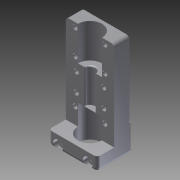
# Autodesk Inventor part: Z move left
Saved by Autodesk Inventor 2012 (Build 160160000, 160)
## iProperties
Created: 2013-02-04
Part Number: Z move left
Material: Default
Document SubType Name: Modeling
Designer: mce
Density: 1 g/cm^3
Mass: 50.5221 g
Surface Area: 165.701 cm^2
Volume: 50.5221 cm^3
Author: mce
Autodesk Inventor part; units mm, degrees
ref_plane "YZ Plane" through (0, 0, 0) normal (1, 0, 0) x (0, 1, 0)
ref_plane "XZ Plane" through (0, 0, 0) normal (0, 1, 0) x (-1, 0, 0)
ref_plane "XY Plane" through (0, 0, 0) normal (0, 0, 1) x (1, 0, 0)
sketch "Sketch1" plane through (0, 0, 0) normal (0, 0, 1) x (1, 0, 0)
  line L0 (0, 0) -> (42.4, 0)
  line L1 (42.4, 0) -> (42.4, 30)
  line L2 (42.4, 30) -> (0, 30)
  line L3 (0, 30) -> (0, 0)
  circle A0 centre (21.2, 15) radius 4.5
  dimension "d0" = 42.4
  dimension "d1" = 30
  dimension "d2" = 21.2
  dimension "d3" = 15
  dimension "d4" = 9
  constraints: 8 end point, 2 horizontal, 2 vertical, 1 centre point
  measures "d0" distance of L0.start L0.end
  measures "d1" distance of L2.end L0.start
  measures "d2" distance from line of L3 A0.centre
  measures "d3" distance from line of L0 A0.centre
  measures "d4" diameter of A0
extrude "Extrusion1" add sketch "Sketch1" along normal blind 90
sketch "Sketch2" plane through (0, 0, 90) normal (0, 0, 1) x (1, 0, 0)
  circle A0 centre (21.2, 15) radius 4.5 projected
  circle A1 centre (21.2, 15) radius 10.5
  dimension "d7" = 21
  constraints: 1 centre point, 1 coincident
  measures "d7" diameter of A1
sketch "Sketch3" plane through (0, 0, 0) normal (0, 0, -1) x (-1, 0, 0)
  circle A0 centre (-21.2, 15) radius 4.5 projected
  circle A1 centre (-21.2, 15) radius 10.5
  dimension "d8" = 21
  constraints: 1 centre point, 1 coincident
  measures "d8" diameter of A1
extrude "Extrusion2" cut sketch "Sketch2" against normal blind 30
sketch "Sketch4" plane through (0, 0, 0) normal (0, -1, 0) x (1, 0, 0)
  line L0 (0, 0) -> (42.4, 0) projected
  line L1 (42.4, 0) -> (42.4, 90) projected
  line L2 (0, 90) -> (42.4, 90)
  line L3 (42.4, 90) -> (42.4, 12)
  line L4 (42.4, 12) -> (0, 12)
  line L5 (0, 12) -> (0, 90)
  dimension "d11" = 12
  constraints: 8 end point, 1 point on line
  measures "d11" distance between parallel lines of L4 L0
extrude "Extrusion3" cut sketch "Sketch4" against normal blind 15
extrude "Extrusion4" cut sketch "Sketch3" against normal blind 30
sketch "Sketch5" plane through (0, 0, 0) normal (0, -1, 0) x (1, 0, 0)
  line L0 (0, 0) -> (42.4, 0) projected
  circle A0 centre (8.2, 4) radius 2.1
  circle A1 centre (34.2, 4) radius 2.1
  circle A2 centre (34.2, 26) radius 2.1
  circle A3 centre (8.2, 26) radius 2.1
  circle A4 centre (8.2, 86) radius 2.1
  circle A5 centre (8.2, 64) radius 2.1
  circle A6 centre (34.2, 86) radius 2.1
  circle A7 centre (34.2, 64) radius 2.1
  line L1 (0, 12) -> (0, 90) projected
  line L2 (8.2, 75.2078) -> (8.2, -13.8243) construction
  line L3 (34.2, 77.256) -> (34.2, -15.4673) construction
  line L4 (42.4, 90) -> (42.4, 12) construction
  line L5 (0, 90) -> (10.7, 90) construction
  line L6 (31.7, 90) -> (42.4, 90) construction
  dimension "d16" = 4.2
  dimension "d18" = 8.2
  dimension "d19" = 4
  dimension "d20" = 22
  dimension "d21" = 4
  dimension "d22" = 22
  dimension "d23" = 8.2
  dimension "d24" = 4
  dimension "d25" = 22
  dimension "d26" = 4
  dimension "d27" = 22
  constraints: 8 centre point, 8 point on line, 7 equal radius, 4 end point, 1 vertical
  measures "d16" diameter of A4
  measures "d18" distance between parallel lines of L3 L4
  measures "d19" distance from line of A4.centre L5
  measures "d20" distance of A4.centre A5.centre
  measures "d21" distance from line of L6 A6.centre
  measures "d22" distance of A7.centre A6.centre
  measures "d23" distance between parallel lines of L1 L2
  measures "d24" distance from line of L0 A0.centre
  measures "d25" distance of A3.centre A0.centre
  measures "d26" distance from line of L0 A1.centre
  measures "d27" distance of A2.centre A1.centre
extrude "Extrusion5" cut sketch "Sketch5" against normal through all
sketch "Sketch6" plane through (0, 30, 0) normal (0, 1, 0) x (1, 0, 0)
  circle A0 centre (34.2, -64) radius 2.1 projected
  circle A1 centre (34.2, -86) radius 2.1 projected
  circle A2 centre (8.2, -64) radius 2.1 projected
  circle A3 centre (8.2, -86) radius 2.1 projected
  line L0 (12.2992, -64) -> (10.2496, -67.55)
  line L1 (10.2496, -67.55) -> (6.1504, -67.55)
  line L2 (6.1504, -67.55) -> (4.1008, -64)
  line L3 (4.1008, -64) -> (6.1504, -60.45)
  line L4 (6.1504, -60.45) -> (10.2496, -60.45)
  line L5 (10.2496, -60.45) -> (12.2992, -64)
  line L6 (38.2992, -64) -> (36.2496, -67.55)
  line L7 (36.2496, -67.55) -> (32.1504, -67.55)
  line L8 (32.1504, -67.55) -> (30.1008, -64)
  line L9 (30.1008, -64) -> (32.1504, -60.45)
  line L10 (32.1504, -60.45) -> (36.2496, -60.45)
  line L11 (36.2496, -60.45) -> (38.2992, -64)
  line L12 (38.2992, -86) -> (36.2496, -89.55)
  line L13 (36.2496, -89.55) -> (32.1504, -89.55)
  line L14 (32.1504, -89.55) -> (30.1008, -86)
  line L15 (30.1008, -86) -> (32.1504, -82.45)
  line L16 (32.1504, -82.45) -> (36.2496, -82.45)
  line L17 (36.2496, -82.45) -> (38.2992, -86)
  line L18 (12.2992, -86) -> (10.2496, -89.55)
  line L19 (10.2496, -89.55) -> (6.1504, -89.55)
  line L20 (6.1504, -89.55) -> (4.1008, -86)
  line L21 (4.1008, -86) -> (6.1504, -82.45)
  line L22 (6.1504, -82.45) -> (10.2496, -82.45)
  line L23 (10.2496, -82.45) -> (12.2992, -86)
  point P0 (8.2, -89.55)
  dimension "d30" = 7.1
  constraints: 48 end point, 4 coincident, 4 horizontal, 3 equal length, 1 midpoint, 52 other
  measures "d30" distance between parallel lines of L22 L19
extrude "Extrusion6" cut sketch "Sketch6" against normal blind 7
sketch "Sketch7" plane through (0, 0, 0) normal (0, -1, 0) x (1, 0, 0)
  circle A0 centre (34.2, 4) radius 2.1 projected
  circle A1 centre (8.2, 4) radius 2.1 projected
  circle A2 centre (8.2, 4) radius 4.25
  circle A3 centre (34.2, 4) radius 4.25
  dimension "d33" = 8.5
  constraints: 2 centre point, 2 coincident, 1 equal radius
  measures "d33" diameter of A2
extrude "Extrusion7" cut sketch "Sketch7" against normal blind 4
fillet "Fillet1" radius 3 1 edges at (42.4, 15, 0)
sketch "Sketch8" plane through (0, 30, 90) normal (0, 1, 0) x (1, 0, 0)
  line L0 (39.4, 90) -> (0, 90) projected
  line L1 (42.4, 87) -> (42.4, 0) projected
  line L2 (10.2496, 7.55) -> (12.2992, 4) projected
  line L3 (12.2992, 4) -> (10.2496, 0.45) projected
  line L4 (10.2496, 0.45) -> (6.1504, 0.45) projected
  line L5 (6.1504, 0.45) -> (4.1008, 4) projected
  line L6 (4.1008, 4) -> (6.1504, 7.55) projected
  line L7 (6.1504, 7.55) -> (10.2496, 7.55) projected
  line L8 (10.2496, 29.55) -> (12.2992, 26) projected
  line L9 (12.2992, 26) -> (10.2496, 22.45) projected
  line L10 (10.2496, 22.45) -> (6.1504, 22.45) projected
  line L11 (6.1504, 22.45) -> (4.1008, 26) projected
  line L12 (4.1008, 26) -> (6.1504, 29.55) projected
  line L13 (6.1504, 29.55) -> (10.2496, 29.55) projected
  line L14 (36.2496, 29.55) -> (38.2992, 26) projected
  line L15 (38.2992, 26) -> (36.2496, 22.45) projected
  line L16 (36.2496, 22.45) -> (32.1504, 22.45) projected
  line L17 (32.1504, 22.45) -> (30.1008, 26) projected
  line L18 (30.1008, 26) -> (32.1504, 29.55) projected
  line L19 (32.1504, 29.55) -> (36.2496, 29.55) projected
  line L20 (36.2496, 7.55) -> (38.2992, 4) projected
  line L21 (38.2992, 4) -> (36.2496, 0.45) projected
  line L22 (36.2496, 0.45) -> (32.1504, 0.45) projected
  line L23 (32.1504, 0.45) -> (30.1008, 4) projected
  line L24 (30.1008, 4) -> (32.1504, 7.55) projected
  line L25 (32.1504, 7.55) -> (36.2496, 7.55) projected
  line L26 (0, 0) -> (42.4, 0)
  line L27 (42.4, 0) -> (42.4, 66)
  line L28 (42.4, 66) -> (0, 66)
  line L29 (0, 66) -> (0, 0)
  dimension "d38" = 24
  constraints: 8 end point, 1 point on line
  measures "d38" distance between parallel lines of L0 L28
extrude "Extrusion8" cut sketch "Sketch8" against normal blind 1
fillet "Fillet2" radius 3 1 edges at (0, 15, 0)
fillet "Fillet3" radius 3 7 edges at (37.5181, 0, 0) (41.5213, 0, 0.8787) (42.4, 0, 7.5) (21.2, 0, 0) (0.8787, 0, 0.8787) (0, 0, 7.5) (4.8819, 0, 0)
fillet "Fillet4" radius 1 12 edges at (0, 29, 57) (21.2, 29, 90) (0.8787, 30, 0.8787) (21.2, 30, 0) (41.5213, 30, 0.8787) (42.4, 30, 13.5) (0, 30, 13.5) (42.4, 29, 57) (21.2, 19.5, 60) (21.2, 19.5, 30) (25.7, 15, 45) (16.7, 15, 45)
sketch "Sketch9" plane through (0, 0, 30) normal (0, 0, -1) x (-1, 0, 0)
  arc A0 (-15.7, 15) -> (-26.7, 15) centre (-21.2, 15) ccw projected
  arc A1 (-10.7, 15) -> (-31.7, 15) centre (-21.2, 15) ccw projected
  arc A2 (-15.7, 15) -> (-26.7, 15) centre (-21.2, 15) ccw
  line L0 (-31.7, 15) -> (-10.7, 15)
  point P0 (0, 0)
  constraints: 2 end point, 2 point on circle, 2 point on line, 1 centre point, 1 coincident, 1 concentric
extrude "Extrusion9" add sketch "Sketch9" against normal blind 0.2 contours L0 A0
fillet "Fillet5" radius 3 4 edges at (0, 21.5, 90) (0.2929, 28.7071, 89.7071) (42.1071, 28.7071, 89.7071) (42.4, 21.5, 90)
sketch "Sketch11" plane through (0, 29, 90) normal (0, 1, 0) x (1, 0, 0)
  circle A0 centre (9.2, 53) radius 2.1
  circle A1 centre (33.2, 53) radius 2.1
  circle A2 centre (33.2, 37) radius 2.1
  circle A3 centre (9.2, 37) radius 2.1
  line L0 (0, 66) -> (0, 3) projected
  line L1 (39.4, 90) -> (3, 90) projected
  line L2 (42.4, 3) -> (42.4, 66) projected
  point P0 (0, 90)
  point P1 (0, 67)
  point P2 (42.4, 67)
  dimension "d55" = 4.2
  dimension "d56" = 9.2
  dimension "d57" = 37
  dimension "d58" = 16
  dimension "d59" = 9.2
  constraints: 4 centre point, 3 equal radius, 2 horizontal alignment, 2 vertical alignment
  measures "d55" diameter of A0
  measures "d56" distance from line of L0 A0.centre
  measures "d57" distance from line of L1 A0.centre
  measures "d58" distance of A0.centre A3.centre
  measures "d59" distance from line of L2 A1.centre
extrude "Extrusion11" cut sketch "Sketch11" against normal through all
sketch "Sketch12" plane through (0, 29, 90) normal (0, 1, 0) x (1, 0, 0)
  circle A0 centre (9.2, 37) radius 2.1 projected
  circle A1 centre (33.2, 37) radius 2.1 projected
  circle A2 centre (33.2, 53) radius 2.1 projected
  circle A3 centre (9.2, 53) radius 2.1 projected
  line L0 (10.2496, 29.55) -> (6.1504, 29.55) projected
  line L1 (13.2992, 53) -> (11.2496, 49.45)
  line L2 (11.2496, 49.45) -> (7.1504, 49.45)
  line L3 (7.1504, 49.45) -> (5.1008, 53)
  line L4 (5.1008, 53) -> (7.1504, 56.55)
  line L5 (7.1504, 56.55) -> (11.2496, 56.55)
  line L6 (11.2496, 56.55) -> (13.2992, 53)
  line L7 (37.2992, 53) -> (35.2496, 49.45)
  line L8 (35.2496, 49.45) -> (31.1504, 49.45)
  line L9 (31.1504, 49.45) -> (29.1008, 53)
  line L10 (29.1008, 53) -> (31.1504, 56.55)
  line L11 (31.1504, 56.55) -> (35.2496, 56.55)
  line L12 (35.2496, 56.55) -> (37.2992, 53)
  line L13 (37.2992, 37) -> (35.2496, 33.45)
  line L14 (35.2496, 33.45) -> (31.1504, 33.45)
  line L15 (31.1504, 33.45) -> (29.1008, 37)
  line L16 (29.1008, 37) -> (31.1504, 40.55)
  line L17 (31.1504, 40.55) -> (35.2496, 40.55)
  line L18 (35.2496, 40.55) -> (37.2992, 37)
  line L19 (13.2992, 37) -> (11.2496, 33.45)
  line L20 (11.2496, 33.45) -> (7.1504, 33.45)
  line L21 (7.1504, 33.45) -> (5.1008, 37)
  line L22 (5.1008, 37) -> (7.1504, 40.55)
  line L23 (7.1504, 40.55) -> (11.2496, 40.55)
  line L24 (11.2496, 40.55) -> (13.2992, 37)
  point P0 (0, 90)
  constraints: 48 end point, 4 coincident, 4 equal length, 4 horizontal, 52 other
extrude "Extrusion12" cut sketch "Sketch12" against normal blind 6
sketch "Sketch10" plane through (42.4, 3, 12) normal (1, 0, 0) x (0, 0, -1)
  circle A0 centre (-49, 20) radius 3
  circle A1 centre (-17, 20) radius 3
  line L0 (-78, 25) -> (-78, 12) projected
  line L1 (12, 0) -> (12, 26) projected
  line L2 (-75, 26) -> (-12, 26) projected
  point P0 (12, -3)
  dimension "d47" = 6
  dimension "d48" = 29
  dimension "d49" = 29
  dimension "d52" = 6
  dimension "d53" = 6
  constraints: 2 centre point, 1 equal radius
  measures "d47" diameter of A0
  measures "d48" distance from line of L0 A0.centre
  measures "d49" distance from line of A1.centre L1
  measures "d52" distance from line of L2 A0.centre
  measures "d53" distance from line of L2 A1.centre
equation "\"d18\" = d23"
equation "\"d22\" = d20"
equation "\"d27\" = d25"
body "Solid1"
